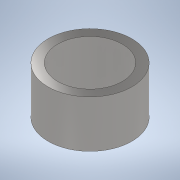
# Autodesk Inventor part: МПСТ Распорная втулка промежуточного вала
Saved by Autodesk Inventor 2022.1 (Build 261234020, 234B)
## iProperties
Created: 2021-12-16
Part Number: МПСТ Распорная втулка промежуточного вала
Material: Сталь, углеродистая
Document SubType Name: Modeling
Designer: Алексанян Г.
Density: 7.85 g/cm^3
Appearance: С умеренной полировкой
Author: Алексанян Г.
Autodesk Inventor part; units mm, degrees
ref_plane "YZ Plane" through (0, 0, 0) normal (1, 0, 0) x (0, 1, 0)
ref_plane "XZ Plane" through (0, 0, 0) normal (0, 1, 0) x (-1, 0, 0)
ref_plane "XY Plane" through (0, 0, 0) normal (0, 0, 1) x (1, 0, 0)
sketch "Эскиз1" plane through (0, 0, 0) normal (0, 0, 1) x (1, 0, 0)
  line L0 (0, 28.9289) -> (0, -27.0571)
  line L1 (-55, 31) -> (-42.5, 31)
  line L2 (-42.5, 31) -> (-42.5, -31)
  line L3 (-42.5, -31) -> (-55, -31)
  line L4 (-55, -31) -> (-55, 31)
  line L5 (-55, 31) -> (-42.5, -31) construction
  line L6 (-42.5, 31) -> (-55, -31) construction
  point P0 (0, 0)
  point P1 (-48.75, 0)
  point P2 (-48.75, 0)
  dimension "d0" = 85
  dimension "d1" = 62
  dimension "d2" = 110
  constraints: 14 end point, 3 midpoint, 2 parallel, 1 horizontal, 1 horizontal alignment, 1 perpendicular, 1 point on line, 1 vertical
  measures "d0" diameter of L2 L0
  measures "d1" distance of L3.end L1.start
  measures "d2" diameter of L4 L0
revolve "Вращение1" add sketch "Эскиз1" angle 360 about axis through (0, 28.9289, 0) along (0, -1, 0)
